finger box_v12 (Autodesk Fusion 360 design; units mm, degrees)
Autodesk Fusion 360 part; units mm, degrees
sketch "Bottom panel sketch" plane through (0, 0, 0) normal (0, 0, 1) x (1, 0, 0)
  line L0 (0, 0) -> (100, 0)
  line L1 (100, 0) -> (100, 75)
  line L2 (100, 75) -> (0, 75)
  line L3 (0, 75) -> (0, 0)
  dimension "d11" = 100
  dimension "d12" = 75
  constraint horizontal L0
  constraint vertical L1
  constraint horizontal L2
  constraint vertical L3
  constraint coincident L0.start L3.end
  measures "d11" distance of L0.start L0.end
  measures "d12" distance of L0.start L2.end
extrude "Extrude1" add sketch "Bottom panel sketch" along normal blind 3.175 makes body 1
sketch "Bottom Panel Front Fingers Sketch" plane through (0, 0, 0) normal (0, -1, 0) x (1, 0, 0)
  line L0 (0, 0) -> (100, 0)
  line L1 (100, 0) -> (100, 3.175)
  line L2 (100, 3.175) -> (0, 3.175)
  line L3 (0, 3.175) -> (0, 0)
  line L4 (9.0909, 0) -> (18.1818, 0)
  line L5 (18.1818, 0) -> (18.1818, 3.175)
  line L6 (18.1818, 3.175) -> (9.0909, 3.175)
  line L7 (9.0909, 3.175) -> (9.0909, 0)
  dimension "d15" = 9.0909
  dimension "d16" = 9.0909
  constraint horizontal L4
  constraint vertical L5
  constraint horizontal L6
  constraint vertical L7
  constraint coincident L0 L4.start
  constraint collinear L2 L6
  measures "d15" distance of L4.start L4.end
  measures "d16" distance of L0.start L4.start
extrude "Extrude2" cut sketch "Bottom Panel Front Fingers Sketch" against normal blind 3.175 contours L0 L2 L4 L5 L6 L7 bodies 1
pattern_linear "R-Pattern1" count 5 spacing 18.1818 along (1, 0, 0) of "Extrude2"
sketch "Front Panel" plane through (0, 0, 0) normal (0, 1, 0) x (1, 0, 0)
  line L0 (0, 0) -> (100, 0)
  line L1 (100, 0) -> (100, -30)
  line L2 (100, -30) -> (0, -30)
  line L3 (0, -30) -> (0, 0)
  point P0 (100, 0)
  dimension "d32" = 30
  constraint perpendicular L0 L1
  constraint parallel L0 L2
  constraint parallel L1 L3
  constraint horizontal L0
  constraint coincident L0.start L3.end
  constraint coincident P0 L0.end
  measures "d32" distance of L0.start L2.end
extrude "Extrude3" add sketch "Front Panel" along normal blind 3.175 separate body makes body 2
combine "Combine1" operation cut target body 2 tool bodies 1 keep tools
sketch "Front Panel Left Fingers" plane through (0, 0, 0) normal (-1, 0, 0) x (0, -1, 0)
  line L0 (-3.175, 3.175) -> (0, 3.175)
  line L1 (0, 3.175) -> (0, 30)
  line L2 (0, 30) -> (-3.175, 30)
  line L3 (-3.175, 30) -> (-3.175, 3.175)
  line L4 (0, 6) -> (0, 12)
  line L5 (0, 12) -> (-3.175, 12)
  line L6 (-3.175, 12) -> (-3.175, 6)
  line L7 (-3.175, 6) -> (0, 6)
  dimension "d35" = 6
  dimension "d36" = 6
  constraint perpendicular L4 L5
  constraint parallel L4 L6
  constraint parallel L5 L7
  constraint coincident L1 L4.end
  constraint parallel L1 L4
  measures "d35" distance of L4.start L4.end
  measures "d36" distance of origin L7
extrude "Extrude4" cut sketch "Front Panel Left Fingers" against normal blind 3.175 contours L1 L3 L4 L5 L6 L7 bodies 2
pattern_linear "R-Pattern3" count 2 spacing 12 along (0, 0, 1) of "Extrude4"
sketch "Bottom Panel Left Fingers Sketch" plane through (0, 0, 0) normal (-1, 0, 0) x (0, -1, 0)
  line L0 (-75, 0) -> (0, 0)
  line L1 (0, 0) -> (0, 3.175)
  line L2 (0, 3.175) -> (-75, 3.175)
  line L3 (-75, 3.175) -> (-75, 0)
  line L4 (-10.7143, 0) -> (-21.4286, 0)
  line L5 (-21.4286, 0) -> (-21.4286, 3.175)
  line L6 (-21.4286, 3.175) -> (-10.7143, 3.175)
  line L7 (-10.7143, 3.175) -> (-10.7143, 0)
  dimension "d43" = 10.7143
  dimension "d44" = 10.7143
  constraint horizontal L4
  constraint vertical L5
  constraint horizontal L6
  constraint vertical L7
  constraint coincident L2 L5.end
  constraint coincident L0 L4.start
  measures "d43" distance of L4.start L4.end
  measures "d44" distance of L1 L7
extrude "Extrude5" cut sketch "Bottom Panel Left Fingers Sketch" against normal blind 3.175 contours L0 L2 L4 L5 L6 L7 bodies 1
pattern_linear "R-Pattern4" count 3 spacing 21.4286 along (0, 1, 0) of "Extrude5"
extrude "Extrude6" add 1 faces at (51.5152, 3.175, 21.0583) along direction (0, -1, 0) blind 3.175 from surface at -71.825 separate body on bodies 2 makes body 3
combine "Combine2" operation cut target body 1 tool bodies 3 keep tools
sketch "Left Panel Sketch" plane through (0, 0, 0) normal (1, 0, 0) x (0, 1, 0)
  line L0 (0, 0) -> (75, 0)
  line L1 (75, 0) -> (75, 30)
  line L2 (75, 30) -> (0, 30)
  line L3 (0, 30) -> (0, 0)
  dimension "d58" = 75
  dimension "d59" = 30
  constraint perpendicular L0 L1
  constraint parallel L0 L2
  constraint parallel L1 L3
  constraint horizontal L0
  constraint coincident L0.start L3.end
  measures "d58" distance of L0.start L0.end
  measures "d59" distance of L0.end L1.end
extrude "Extrude7" add sketch "Left Panel Sketch" along normal blind 3.175 separate body makes body 4
combine "Combine4" operation cut target body 4 tool bodies 3 2 1 keep tools
copy_body "CopyPasteBodies2" bodies 4 makes body 5
move_body "Move2" bodies 5 to x (1, 0, 0) y (0, 1, 0) z (0, 0, 1) at (96.825, 0, 0)
combine "Combine7" operation cut target body 2 tool bodies 5 keep tools
combine "Combine8" operation cut target body 1 tool bodies 5 keep tools
combine "Combine9" operation cut target body 3 tool bodies 5 keep tools
equation "length = 100 mm"
equation "width = 75 mm"
equation "height = 30 mm"
equation "thickness = 3.175 mm"
equation "lFingerW = length / ( lFingers * 2 + 1 )"
equation "wFingerW = width / ( wFingers * 2 + 1 )"
equation "hFingerW = height / ( hFingers * 2 + 1 )"
equation "d11 = length"
equation "d12 = width"
equation "d13 = thickness"
equation "d15 = lFingerW"
equation "d16 = lFingerW"
equation "d17 = -thickness"
equation "d19 = lFingers"
equation "d21 = length - lFingerW * 3"
equation "lFingers = 5"
equation "wFingers = 3"
equation "hFingers = 2"
equation "d32 = height"
equation "d33 = thickness"
equation "d35 = hFingerW"
equation "d36 = hFingerW"
equation "d37 = -thickness"
equation "d39 = hFingers"
equation "d41 = -height + hFingerW * 3"
equation "d43 = wFingerW"
equation "d44 = wFingerW"
equation "d45 = -thickness"
equation "d47 = wFingers"
equation "d49 = -width + 3 * wFingerW"
equation "d56 = -thickness"
equation "d58 = width"
equation "d59 = height"
equation "d60 = thickness"
equation "d70 = length - thickness"
named bodies: "Bottom panel", "Front panel", "Back panel", "Left Panel", "Left Panel (1)"
